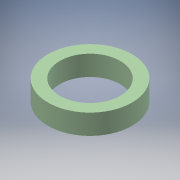
# Autodesk Inventor part: FoilCoil3
Saved by Autodesk Inventor 2019 (Build 230136000, 136)
## iProperties
Created: 2017-01-18
Part Number: FoilCoil3
Document SubType Name: Modeling
Designer: Administrator
Density: 1 g/cm^3
Mass: 1.41843 g
Surface Area: 12.8334 cm^2
Volume: 1.41843 cm^3
Material: Generic
Appearance: Green Pastel
Author: Administrator
Autodesk Inventor part; units mm, degrees
ref_plane "YZ Plane" through (0, 0, 0) normal (1, 0, 0) x (0, 1, 0)
ref_plane "XZ Plane" through (0, 0, 0) normal (0, 1, 0) x (-1, 0, 0)
ref_plane "XY Plane" through (0, 0, 0) normal (0, 0, 1) x (1, 0, 0)
sketch "Sketch4" plane through (0, 0, 0) normal (0, 0, 1) x (1, 0, 0)
  circle A0 centre (0, 0) radius 9
  circle A1 centre (0, 0) radius 12.5
  dimension "d9" = 18
  dimension "d10" = 25
  constraints: 2 centre point, 1 other
  measures "d9" diameter of A0
  measures "d10" diameter of A1
extrude "Extrusion4" add sketch "Sketch4" along normal mid plane 6
body "Solid1"
